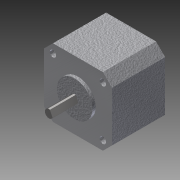
# Autodesk Inventor part: stepper42BYGH007_RB01
Saved by Autodesk Inventor 2013 (Build 170138000, 138)
## iProperties
Created: 2014-06-13
Part Number: stepper42BYGH007_RB01
Material: Aluminum-6061
Document SubType Name: Modeling
Designer: Byron
Density: 2.71 g/cm^3
Mass: 152.548 g
Surface Area: 105.247 cm^2
Volume: 56.2907 cm^3
Author: Byron
Autodesk Inventor part; units mm, degrees
ref_plane "YZ Plane" through (0, 0, 0) normal (1, 0, 0) x (0, 1, 0)
ref_plane "XZ Plane" through (0, 0, 0) normal (0, 1, 0) x (-1, 0, 0)
ref_plane "XY Plane" through (0, 0, 0) normal (0, 0, 1) x (1, 0, 0)
sketch "Sketch1" plane through (0, 0, 0) normal (0, 0, 1) x (1, 0, 0)
  line L0 (5.6515, 0) -> (36.6485, 0)
  line L1 (42.3, 5.6515) -> (42.3, 36.6485)
  line L2 (36.6485, 42.3) -> (5.6515, 42.3)
  line L3 (0, 36.6485) -> (0, 5.6515)
  line L4 (0, 36.6485) -> (5.6515, 42.3)
  line L5 (36.6485, 42.3) -> (42.3, 36.6485)
  line L6 (42.3, 5.6515) -> (36.6485, 0)
  line L7 (5.6515, 0) -> (0, 5.6515)
  line L8 (21.15, 42.3) -> (21.15, 0) construction
  line L9 (0, 21.9578) -> (42.3, 21.9578) construction
  point P0 (0, 0)
  point P1 (42.3, 42.3)
  point P2 (42.3, 0)
  point P3 (0, 42.3)
  dimension "d0" = 42.3
  dimension "d1" = 42.3
  dimension "d2" = 5.6515
  dimension "d3" = 5.6515
  dimension "d4" = 5.6515
  dimension "d5" = 5.6515
  dimension "d6" = 5.6515
  dimension "d7" = 5.6515
  dimension "d8" = 5.6515
  dimension "d9" = 5.6515
  dimension "d10" = 30.997
  constraints: 20 end point, 10 point on line, 2 midpoint, 2 parallel, 2 perpendicular, 1 horizontal
  measures "d0" distance of point (0, 42.3) point (42.3, 42.3)
  measures "d1" distance of point (42.3, 42.3) point (42.3, 0)
  measures "d2" distance of L3.start point (0, 42.3)
  measures "d3" distance of L2.end point (0, 42.3)
  measures "d4" distance of L2.start point (42.3, 42.3)
  measures "d5" distance of L1.end point (42.3, 42.3)
  measures "d6" distance of L1.start point (42.3, 0)
  measures "d7" distance of L0.end point (42.3, 0)
  measures "d8" distance of L0.start point (0, 0)
  measures "d9" distance of L3.end point (0, 0)
  measures "d10" distance of L3.start L3.end
extrude "Extrusion1" add sketch "Sketch1" along normal blind 33.02
sketch "Sketch2" plane through (0, 0, 33.02) normal (0, 0, 1) x (1, 0, 0)
  line L0 (5.6515, 42.3) -> (36.6485, 42.3) projected
  line L1 (0, 5.6515) -> (0, 36.6485) projected
  line L2 (36.6485, 0) -> (5.6515, 0) projected
  line L3 (42.3, 36.6485) -> (42.3, 5.6515) projected
  line L4 (21.15, 42.3) -> (21.15, 0) construction
  line L5 (0, 21.15) -> (42.3, 21.15) construction
  circle A0 centre (21.15, 21.15) radius 11
  point P0 (0, 0)
  dimension "d13" = 22
  constraints: 5 midpoint, 4 end point, 1 centre point
  measures "d13" diameter of A0
extrude "Extrusion2" add sketch "Sketch2" along normal blind 2
sketch "Sketch3" plane through (21.15, 21.15, 35.02) normal (0, 0, 1) x (1, 0, 0)
  circle A0 centre (0, 0) radius 11 projected
  arc A1 (0.6085, 2.4399) -> (2.2645, -1.0932) centre (0, 0) ccw
  line L0 (0.6085, 2.4399) -> (2.2645, -1.0932)
  line L1 (1.4365, 0.6733) -> (-2.2769, -1.0672) construction
  point P0 (-21.15, -21.15)
  dimension "d16" = 5.0292
  dimension "d34" = 3.9019
  dimension "d36" = 1.951
  dimension "d37" = 4.1011
  constraints: 4 end point, 3 point on circle, 1 centre point, 1 coincident, 1 midpoint, 1 perpendicular
  measures "d16" diameter of A1
  measures "d34" distance of L0.start L0.end
  measures "d36" distance of L0.start L1.start
  measures "d37" distance of L1.start L1.end
extrude "Extrusion3" add sketch "Sketch3" along normal blind 16.002 contours L0 A1
sketch "Sketch4" plane through (0, 0, 33.02) normal (0, 0, 1) x (1, 0, 0)
  line L0 (0, 36.6485) -> (5.6515, 42.3) projected
  line L1 (5.6515, 0) -> (0, 5.6515) projected
  line L2 (42.3, 5.6515) -> (36.6485, 0) projected
  line L3 (36.6485, 42.3) -> (42.3, 36.6485) projected
  line L4 (2.8258, 39.4742) -> (39.4742, 2.8258) construction
  line L5 (39.4742, 39.4742) -> (2.8257, 2.8258) construction
  point P0 (0, 0)
  point P1 (5.65, 36.65)
  point P2 (36.65, 36.65)
  point P3 (5.65, 5.65)
  point P4 (36.65, 5.65)
  dimension "d20" = 31
  dimension "d21" = 31
  dimension "d22" = 31
  dimension "d23" = 31
  constraints: 4 end point, 4 midpoint, 4 point on line, 1 perpendicular
  measures "d20" distance of point (36.65, 36.65) point (5.65, 36.65)
  measures "d21" distance of point (5.65, 5.65) point (5.65, 36.65)
  measures "d22" distance of point (36.65, 5.65) point (5.65, 5.65)
  measures "d23" distance of point (36.65, 5.65) point (36.65, 36.65)
hole "Hole1" at (5.65, 36.65, 33.02) at (36.65, 36.65, 33.02) at (5.65, 5.65, 33.02) at (36.65, 5.65, 33.02) direction (0, 0, -1) diameter 4 end through all
equation "\"d3\" = d2"
equation "\"d4\" = d2"
equation "\"d5\" = d4"
equation "\"d6\" = d2"
equation "\"d7\" = d6"
equation "\"d8\" = d2"
equation "\"d9\" = d8"
equation "\"d36\" = 0.5 * d34"
equation "\"d21\" = d20"
equation "\"d22\" = d20"
equation "\"d23\" = d20"
body "Solid1"
